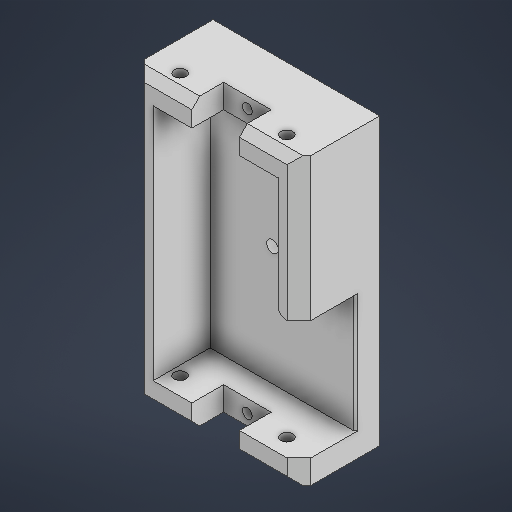
# Autodesk Inventor part: GA_Base
Saved by Autodesk Inventor 2025.2 (Build 292293000, 293)
## iProperties
Created: 2025-06-18
Part Number: GA_Base
Material: Generic
Document SubType Name: Modeling
Designer: Tiago
Density: 1 g/cm^3
Appearance: Default
Author: Tiago
Autodesk Inventor part; units mm, degrees
ref_plane "YZ Plane" through (0, 0, 0) normal (1, 0, 0) x (0, 1, 0)
ref_plane "XZ Plane" through (0, 0, 0) normal (0, 1, 0) x (-1, 0, 0)
ref_plane "XY Plane" through (0, 0, 0) normal (0, 0, 1) x (1, 0, 0)
sketch "Sketch1" plane through (0, 0, 0) normal (0, 0, 1) x (1, 0, 0)
  line L0 (-15.75, 30) -> (15.75, 30)
  line L1 (15.75, 30) -> (15.75, -30)
  line L2 (15.75, -30) -> (-15.75, -30)
  line L3 (-15.75, -30) -> (-15.75, 30)
  line L4 (-21, -36) -> (21, -36)
  line L5 (21, -36) -> (21, 36)
  line L6 (21, 36) -> (-21, 36)
  line L7 (-21, 36) -> (-21, -36)
  circle A0 centre (0, 0) radius 1.5
  point P0 (15.75, 0)
  point P1 (0, 30)
  point P2 (0, 36)
  point P3 (-21, 0)
  dimension "d0" = 31.5
  dimension "d1" = 60
  dimension "d4" = 42
  dimension "d5" = 72
  dimension "d40" = 3
  constraints: 16 end point, 5 coincident, 4 midpoint, 4 parallel, 2 horizontal, 2 horizontal alignment, 2 perpendicular, 2 vertical alignment, 1 centre point
  measures "d0" distance of L1.end L2.end
  measures "d1" distance of L0.end L1.end
  measures "d4" distance of L5.end L6.end
  measures "d5" distance of L4.end L5.end
  measures "d40" diameter of A0
extrude "Extrusion1" add sketch "Sketch1" along normal blind 20.35 contours L7 L6 L5 L4
extrude "Extrusion2" add sketch "Sketch1" along normal blind 6 contours L0 L1 L2 L3
chamfer "Chamfer1" distance 3 angle 45 2 edges at (21, 0, 20.35) (-21, 0, 20.35)
chamfer "Chamfer2" distance 2 angle 45 2 edges at (0, -36, 20.35) (0, 36, 20.35)
sketch "Sketch2" plane through (0, 0, 20.35) normal (0, 0, 1) x (1, 0, 0)
  line L0 (-18, 34) -> (18, 34) projected
  line L1 (18, 34) -> (18, -34) projected
  line L2 (18, -34) -> (-18, -34) projected
  line L3 (-18, -34) -> (-18, 34) projected
  line L4 (15.75, 30) -> (-15.75, 30) projected
  line L5 (-15.75, 30) -> (-15.75, -30) projected
  line L6 (-15.75, -30) -> (15.75, -30) projected
  line L7 (15.75, -30) -> (15.75, 30) projected
  circle A0 centre (0, -33.25) radius 1.25
  line L8 (-6, -38) -> (6, -38)
  line L9 (6, -38) -> (6, -30)
  line L10 (6, -30) -> (-6, -30)
  line L11 (-6, -30) -> (-6, -38)
  line L12 (-3.2097, 0) -> (3.2097, 0) construction
  circle A1 centre (0, 33.25) radius 1.25
  line L13 (-6, 38) -> (6, 38)
  line L14 (6, 38) -> (6, 30)
  line L15 (6, 30) -> (-6, 30)
  line L16 (-6, 30) -> (-6, 38)
  point P0 (0, 0)
  point P1 (0, -30)
  point P2 (0, -30)
  point P3 (0, 0)
  point P4 (0, 30)
  point P5 (0, 30)
  dimension "d16" = 2.5
  dimension "d18" = 33.25
  dimension "d19" = 12
  dimension "d20" = 8
  constraints: 18 end point, 7 symmetric about line, 3 coincident, 3 midpoint, 2 centre point, 2 horizontal, 2 parallel, 2 vertical alignment, 1 perpendicular, 1 other
  measures "d16" diameter of A0
  measures "d18" distance of point (0, 0) A0.centre
  measures "d19" distance between parallel lines of L11 L9
  measures "d20" distance of L8.end L9.end
extrude "Extrusion3" cut sketch "Sketch2" against normal blind 8 contours L16 L13 L14 L0 A1 | L0 A1 L14 L4 L16 | L11 L6 L9 L2 A0 | L2 A0 L9 L8 L11
extrude "Extrusion4" cut sketch "Sketch2" against normal blind 18 contours A1 L0 | L0 A1 | A0 L2 | L2 A0
ref_plane "Work Plane1" through (15.75, -36, 0) normal (1, 0, 0) x (0, 0, -1)
sketch "Sketch4" plane through (15.75, -36, 0) normal (1, 0, 0) x (0, 0, -1)
  line L0 (-18.35, 72) -> (0, 72) projected
  line L1 (0, 72) -> (0, 0) projected
  line L2 (0, 0) -> (-18.35, 0) projected
  line L3 (-18.35, 0) -> (-20.35, 2) projected
  line L4 (-20.35, 2) -> (-20.35, 6) projected
  line L5 (-20.35, 6) -> (-20.35, 66) projected
  line L6 (-20.35, 66) -> (-20.35, 70) projected
  line L7 (-20.35, 70) -> (-18.35, 72) projected
  line L8 (-20.35, 6) -> (-6, 6) projected
  line L9 (-6, 6) -> (-6, 66) projected
  line L10 (-6, 66) -> (-20.35, 66) projected
  line L11 (-20.35, 6) -> (-6, 6)
  line L12 (-6, 6) -> (-6, 36)
  line L13 (-6, 6) -> (-6, 66) projected
  line L14 (-6, 36) -> (-20.35, 36)
  line L15 (-20.35, 36) -> (-20.35, 6)
  point P0 (0, 36)
  dimension "d26" = 30
  constraints: 8 end point, 2 midpoint, 1 collinear, 1 horizontal
  measures "d26" distance of L8.end L12.end
extrude "Extrusion5" cut sketch "Sketch4" along normal up to surface (5.25 mm away) contours L14 L9 L8 L5
fillet "Fillet1" radius 2 1 edges at (15.75, 0, 13.175)
chamfer "Chamfer3" distance 0.5 angle 45 1 edges at (21, -15, 6)
ref_plane "Work Plane2" through (-21, 33, 0) normal (0, 1, 0) x (1, 0, 0)
sketch "Sketch6" plane through (-21, 33, 0) normal (0, 1, 0) x (1, 0, 0)
  line L0 (15, -12.35) -> (15, -20.35) projected
  line L1 (15, -20.35) -> (3, -20.35) projected
  line L2 (3, -20.35) -> (0, -17.35) projected
  line L3 (0, -17.35) -> (0, 0) projected
  line L4 (0, 0) -> (42, 0) projected
  line L5 (42, 0) -> (42, -17.35) projected
  line L6 (42, -17.35) -> (39, -20.35) projected
  line L7 (39, -20.35) -> (27, -20.35) projected
  line L8 (27, -20.35) -> (27, -12.35) projected
  line L9 (27, -12.35) -> (22.2247, -12.35) projected
  line L10 (22.2247, -12.35) -> (22.2247, -2.35) projected
  line L11 (22.2247, -2.35) -> (19.7753, -2.35) projected
  line L12 (19.7753, -2.35) -> (19.7753, -12.35) projected
  line L13 (19.7753, -12.35) -> (15, -12.35) projected
  circle A0 centre (34.45, -15.85) radius 1.5
  circle A1 centre (7.55, -15.85) radius 1.5
  point P0 (21, 0)
  dimension "Veio" = 3
  dimension "d34" = 3
  dimension "d35" = 4.5
  dimension "d36" = 7.55
  dimension "d37" = 7.55
  constraints: 2 centre point, 1 horizontal alignment
  measures "Veio" diameter of A0
  measures "d34" diameter of A1
  measures "d35" distance from line of L7 A0.centre
  measures "d36" distance from line of L5 A0.centre
  measures "d37" distance from line of L3 A1.centre
extrude "Extrusion6" cut sketch "Sketch6" along normal through all both and the other way through all contours A0 | A1
equation "\"d40\" = Veio"
equation "\"d34\" = Veio"
body "Solid1"
